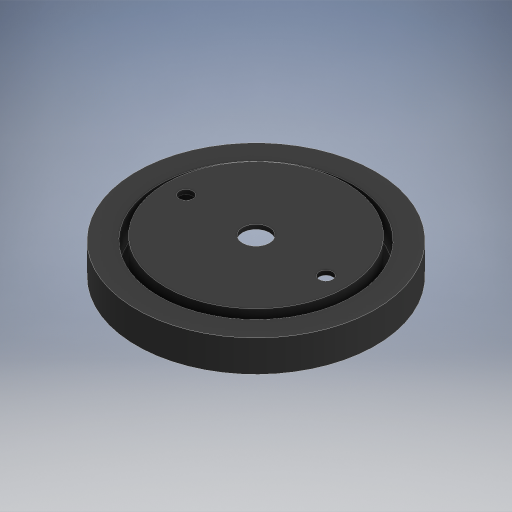
# Autodesk Inventor part: Diaphram
Saved by Autodesk Inventor 2024.1 (Build 281209000, 209)
## iProperties
Created: 2023-11-09
Part Number: Diaphram
Material: Rubber, Silicone
Document SubType Name: Modeling
Designer: Glen Collingwood
Density: 1.25 g/cm^3
Appearance: Rubber - Black
Author: Glen Collingwood
Autodesk Inventor part; units mm, degrees
ref_plane "YZ Plane" through (0, 0, 0) normal (1, 0, 0) x (0, 1, 0)
ref_plane "XZ Plane" through (0, 0, 0) normal (0, 1, 0) x (-1, 0, 0)
ref_plane "XY Plane" through (0, 0, 0) normal (0, 0, 1) x (1, 0, 0)
sketch "Sketch1" plane through (0, 0, 0) normal (1, 0, 0) x (0, 1, 0)
  line L0 (0, 0) -> (-4.0897, 0)
  line L1 (0, -1.6442) -> (0, -13.25)
  line L2 (0, -13.25) -> (3.5, -13.25)
  line L3 (3.5, -13.25) -> (3.5, -10.75)
  line L4 (3.5, -10.75) -> (0.5, -10.75)
  line L5 (4, 0) -> (4, -10)
  line L6 (4, -10) -> (0.5, -10)
  line L7 (0.5, -10) -> (0.5, -10.75)
  line L8 (3.5, -1.5) -> (3.5, -9.5)
  line L9 (3.5, -9.5) -> (0, -9.5)
  line L10 (3, -11.25) -> (0, -11.25)
  line L11 (3, -11.25) -> (3, -12.25)
  line L12 (3, -12.25) -> (0, -12.25)
  line L13 (3.5, -1.5) -> (4, -1.5)
  point P0 (1.5, -12.25)
  point P1 (3.75, -1.5)
  dimension "d1" = 26.5
  dimension "d2" = 2.5
  dimension "d3" = 3.5
  dimension "d4" = 0
  dimension "d5" = 4
  dimension "d6" = 20
  dimension "d7" = 0.5
  dimension "d8" = 0.5
  dimension "d9" = 0.5
  dimension "d10" = 0.5
  dimension "d11" = 0.5
  dimension "d12" = 1
  dimension "d13" = 3
  constraints: 28 end point, 9 perpendicular, 4 point on line, 3 vertical, 2 midpoint, 1 coincident, 1 horizontal
  measures "d1" diameter of L2 L0
  measures "d2" distance of L2.end L3.end
  measures "d3" distance of L1.end L2.end
  measures "d4" distance from line of point (0, 0) L1
  measures "d5" distance between parallel lines of L1 L5
  measures "d6" diameter of L6 L0
  measures "d7" distance between parallel lines of L1 L7
  measures "d8" distance between parallel lines of L6 L9
  measures "d9" distance between parallel lines of L5 L8
  measures "d10" distance between parallel lines of L4 L10
  measures "d11" distance between parallel lines of L3 L11
  measures "d12" distance from line of L2 point (1.5, -12.25)
  measures "d13" diameter of point (3.75, -1.5) L0
revolve "Revolution1" add sketch "Sketch1" angle 360 about axis through (0, 0, 0) along (0, -1, 0) contours L9 L8 L13 L5 L6 L7 L4 L3 L2 L1 L12 L11 L10
sketch "Sketch2" plane through (0, 4, 0) normal (0, 1, 0) x (1, 0, 0)
  line L0 (-7.75, 0) -> (7.75, 0)
  point P0 (0, 0)
  point P1 (0, 0)
  dimension "d15" = 15.5
  constraints: 2 end point, 1 coincident, 1 horizontal, 1 midpoint
  measures "d15" distance of L0.start L0.end
hole "Hole1" at (-7.75, 4, 0) at (7.75, 4, 0) direction (0, -1, 0) diameter 1.5 end through all
fillet "Fillet1" radius 0.6 2 edges at (0, 0, 11.25) (0, 0, 9.5)
equation "\"d8\" = d7"
equation "\"d9\" = d7"
equation "\"d10\" = d7"
equation "\"d11\" = d7"
body "Solid1"
